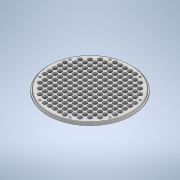
# Autodesk Inventor part: fanCover
Saved by Autodesk Inventor 2021 (Build 250183000, 183)
## iProperties
Created: 2021-04-02
Part Number: fanCover
Material: Generic
Document SubType Name: Modeling
Designer: awitc
Density: 1 g/cm^3
Appearance: Default
Author: awitc
Autodesk Inventor part; units mm, degrees
ref_plane "YZ Plane" through (0, 0, 0) normal (1, 0, 0) x (0, 1, 0)
ref_plane "XZ Plane" through (0, 0, 0) normal (0, 1, 0) x (-1, 0, 0)
ref_plane "XY Plane" through (0, 0, 0) normal (0, 0, 1) x (1, 0, 0)
sketch "Sketch1" plane through (0, 0, 0) normal (0, 1, 0) x (-1, 0, 0)
  circle A0 centre (0, 0) radius 42
  circle A1 centre (0, 0) radius 41
  dimension "d0" = 84
  dimension "d1" = 82
  constraints: 2 centre point, 2 coincident
  measures "d0" diameter of A0
  measures "d1" diameter of A1
extrude "Extrusion1" add sketch "Sketch1" along normal blind 2.5 contours A1
extrude "Extrusion2" add sketch "Sketch1" along normal blind 1
chamfer "Chamfer1" distance 0.5 angle 45 1 edges at (41, 2.5, 0)
sketch "Sketch2" plane through (0, 2.5, 0) normal (0, 1, 0) x (1, 0, 0)
  circle A0 centre (0, 0) radius 40
  line L0 (0, 0) -> (-35, 0)
  line L1 (-35, 0) -> (-30, 0)
  line L2 (-30, 0) -> (-25, 0)
  line L3 (-25, 0) -> (-20, 0)
  line L4 (-20, 0) -> (-15, 0)
  line L5 (-15, 0) -> (-10, 0)
  line L6 (-10, 0) -> (-5, 0)
  circle A1 centre (-35, 0) radius 2
  circle A2 centre (-30, 0) radius 2
  circle A3 centre (-25, 0) radius 2
  circle A4 centre (-20, 0) radius 2
  circle A5 centre (-15, 0) radius 2
  circle A6 centre (-10, 0) radius 2
  circle A7 centre (-5, 0) radius 2
  circle A8 centre (0, 0) radius 2
  line L7 (0, 0) -> (0, 5)
  line L8 (0, 5) -> (0, 10)
  line L9 (0, 10) -> (0, 15)
  line L10 (0, 15) -> (0, 20)
  line L11 (0, 20) -> (0, 25)
  line L12 (0, 25) -> (0, 30)
  line L13 (0, 30) -> (0, 35)
  line L14 (0, 35) -> (0, 40)
  circle A9 centre (0, 35) radius 2
  circle A10 centre (0, 30) radius 2
  circle A11 centre (0, 25) radius 2
  circle A12 centre (0, 20) radius 2
  circle A13 centre (0, 15) radius 2
  circle A14 centre (0, 10) radius 2
  circle A15 centre (0, 5) radius 2
  circle A16 centre (-5, 5) radius 2
  circle A17 centre (-5, 10) radius 2
  circle A18 centre (-5, 15) radius 2
  circle A19 centre (-5, 20) radius 2
  circle A20 centre (-5, 25) radius 2
  circle A21 centre (-5, 30) radius 2
  circle A22 centre (-5, 35) radius 2
  circle A23 centre (-10, 5) radius 2
  circle A24 centre (-15, 5) radius 2
  circle A25 centre (-20, 5) radius 2
  circle A26 centre (-25, 5) radius 2
  circle A27 centre (-30, 5) radius 2
  circle A28 centre (-35, 5) radius 2
  circle A29 centre (-10, 10) radius 2
  circle A30 centre (-10, 15) radius 2
  circle A31 centre (-10, 20) radius 2
  circle A32 centre (-10, 25) radius 2
  circle A33 centre (-10, 30) radius 2
  circle A34 centre (-10, 35) radius 2
  circle A35 centre (-15, 10) radius 2
  circle A36 centre (-20, 10) radius 2
  circle A37 centre (-25, 10) radius 2
  circle A38 centre (-30, 10) radius 2
  circle A39 centre (-35, 10) radius 2
  circle A40 centre (-15, 15) radius 2
  circle A41 centre (-15, 20) radius 2
  circle A42 centre (-15, 25) radius 2
  circle A43 centre (-15, 30) radius 2
  circle A44 centre (-20, 15) radius 2
  circle A45 centre (-25, 15) radius 2
  circle A46 centre (-30, 15) radius 2
  circle A47 centre (-20, 20) radius 2
  circle A48 centre (-25, 20) radius 2
  circle A49 centre (-20, 25) radius 2
  circle A50 centre (-30, 20) radius 2
  circle A51 centre (-20, 30) radius 2
  circle A52 centre (-25, 25) radius 2
  circle A53 centre (-35, 15) radius 1
  circle A54 centre (-15, 35) radius 1
  dimension "d55" = 35
  dimension "d56" = 5
  dimension "d57" = 5
  dimension "d58" = 5
  dimension "d59" = 5
  dimension "d60" = 5
  dimension "d61" = 5
  dimension "d62" = 4
  dimension "d63" = 4
  dimension "d64" = 4
  dimension "d65" = 4
  dimension "d66" = 4
  dimension "d67" = 4
  dimension "d68" = 4
  dimension "d69" = 4
  dimension "d70" = 5
  dimension "d71" = 5
  dimension "d72" = 5
  dimension "d73" = 5
  dimension "d74" = 5
  dimension "d75" = 5
  dimension "d76" = 5
  dimension "d77" = 5
  dimension "d78" = 4
  dimension "d79" = 4
  dimension "d80" = 4
  dimension "d81" = 4
  dimension "d82" = 4
  dimension "d83" = 4
  dimension "d84" = 4
  dimension "d85" = 4
  dimension "d86" = 4
  dimension "d87" = 4
  dimension "d88" = 4
  dimension "d89" = 4
  dimension "d90" = 4
  dimension "d91" = 4
  dimension "d92" = 4
  dimension "d93" = 4
  dimension "d94" = 4
  dimension "d95" = 4
  dimension "d96" = 4
  dimension "d97" = 4
  dimension "d98" = 4
  dimension "d99" = 4
  dimension "d100" = 4
  dimension "d101" = 4
  dimension "d102" = 4
  dimension "d103" = 4
  dimension "d104" = 4
  dimension "d105" = 4
  dimension "d106" = 4
  dimension "d107" = 4
  dimension "d108" = 4
  dimension "d109" = 4
  dimension "d110" = 4
  dimension "d111" = 4
  dimension "d112" = 4
  dimension "d113" = 4
  dimension "d114" = 4
  dimension "d115" = 4
  dimension "d116" = 4
  dimension "d117" = 4
  dimension "d118" = 4
  constraints: 54 centre point, 30 end point, 15 coincident, 12 point on line, 1 horizontal, 1 vertical, 1 vertical alignment, 2 other
  measures "d55" distance of L0.start L0.end
  measures "d56" distance of L0.end L1.end
  measures "d57" distance of L1.end L2.end
  measures "d58" distance of L2.end L3.end
  measures "d59" distance of L3.end L4.end
  measures "d60" distance of L4.end L5.end
  measures "d61" distance of L5.end L6.end
  measures "d62" diameter of A1
  measures "d63" diameter of A2
  measures "d64" diameter of A3
  measures "d65" diameter of A4
  measures "d66" diameter of A5
  measures "d67" diameter of A6
  measures "d68" diameter of A7
  measures "d69" diameter of A8
  measures "d70" distance of L7.start L7.end
  measures "d71" distance of L7.end L8.end
  measures "d72" distance of L8.end L9.end
  measures "d73" distance of L9.end L10.end
  measures "d74" distance of L10.end L11.end
  measures "d75" distance of L11.end L12.end
  measures "d76" distance of L12.end L13.end
  measures "d77" distance of L13.end L14.end
  measures "d78" diameter of A9
  measures "d79" diameter of A10
  measures "d80" diameter of A11
  measures "d81" diameter of A12
  measures "d82" diameter of A13
  measures "d83" diameter of A14
  measures "d84" diameter of A15
  measures "d85" diameter of A16
  measures "d86" diameter of A17
  measures "d87" diameter of A18
  measures "d88" diameter of A19
  measures "d89" diameter of A20
  measures "d90" diameter of A21
  measures "d91" diameter of A22
  measures "d92" diameter of A23
  measures "d93" diameter of A24
  measures "d94" diameter of A25
  measures "d95" diameter of A26
  measures "d96" diameter of A27
  measures "d97" diameter of A28
  measures "d98" diameter of A29
  measures "d99" diameter of A30
  measures "d100" diameter of A31
  measures "d101" diameter of A32
  measures "d102" diameter of A33
  measures "d103" diameter of A34
  measures "d104" diameter of A35
  measures "d105" diameter of A36
  measures "d106" diameter of A37
  measures "d107" diameter of A38
  measures "d108" diameter of A39
  measures "d109" diameter of A40
  measures "d110" diameter of A41
  measures "d111" diameter of A42
  measures "d112" diameter of A43
  measures "d113" diameter of A44
  measures "d114" diameter of A45
  measures "d115" diameter of A46
  measures "d116" diameter of A47
  measures "d117" diameter of A48
  measures "d118" diameter of A49
extrude "Extrusion5" cut sketch "Sketch2" against normal up to surface (2.5 mm away) contours A1 | A2 L0 | L0 A2 | A3 L0 | L0 A3 | A4 L0 | L0 A4 | A5 L0 | L0 A5 | A6 L0 | L0 A6 | A7 L0 | L0 A7 | A8 L0 L7 | L7 L0 A8 | A15 L7 L8 | L8 L7 A15 | A14 L8 L9 | L9 L8 A14 | A13 L9 L10 | L10 L9 A13 | A12 L10 L11 | L11 L10 A12 | A11 L11 L12 | L12 L11 A11 | A10 L12 L13 | L13 L12 A10 | A9 L13 L14 | L14 L13 A9 | A16 | A17 | A18 | A19 | A20 | A21 | A22 | A23 | A24 | A25 | A26 | A27 | A28 | A29 | A30 | A31 | A32 | A33 | A34 | A35 | A36 | A37 | A38 | A39 | A40 | A41 | A42 | A43 | A44 | A45 | A46 | A47 | A48 | A49 | A50 | A51 | A52 | A53 | A54
mirror "Mirror1" about plane through (0, 0, 0) normal (1, 0, 0) of "Extrusion5"
mirror "Mirror2" about plane through (0, 0, 0) normal (0, 0, 1) of "Extrusion5", "Mirror1"
equation "\"d124\" = d94"
body "Solid1"
